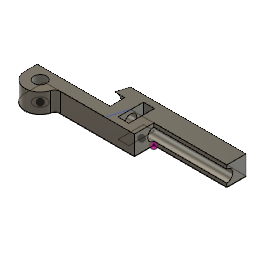
belt-tightener (Autodesk Fusion 360 design; units mm, degrees)
Autodesk Fusion 360 part; units mm, degrees
note: some values were not read from the file. Set by a fixed rule: which sketch regions a step uses.
sketch "Sketch1" plane through (0, 0, 0) normal (0, 1, 0) x (1, 0, 0)
  line L0 (12, 3.2) -> (12, 0)
  line L1 (12, 0) -> (0, 0)
  line L2 (-18, -3.2) -> (-18, 0)
  circle A0 centre (-15.5, -3.2) radius 1.05
  line L3 (-7.0785, 3.2) -> (-8, 0)
  line L4 (-8, 0) -> (-18, 0)
  line L5 (-7.0785, 3.2) -> (12, 3.2)
  line L6 (-3.8, 2.1) -> (-3.8, -2.1)
  line L7 (-3.8, -2.1) -> (-2, -2.1)
  line L8 (-2, -2.1) -> (-2, 2.1)
  line L9 (-2, 2.1) -> (-3.8, 2.1)
  line L10 (0, -3.2) -> (-13, -3.2)
  line L11 (0, -3.2) -> (0, 0)
  arc A1 (-18, -3.2) -> (-13, -3.2) centre (-15.5, -3.2) ccw
  dimension "d9" = 2.1
  dimension "d15" = 3.2
  dimension "d22" = 10
  dimension "d23" = 4.2
  dimension "d24" = 1.8
  dimension "d35" = 12
  dimension "d37" = 2.5
  dimension "d39" = 3.2
  dimension "d40" = 18
  dimension "d42" = 5
  dimension "d43" = 3.2
  dimension "d50" = 2
  measures "d9" diameter of A0
  measures "d35" distance of L1.end
  measures "d37" distance of L2
  measures "d39" distance of L1.end
  measures "d40" distance of L2 L11
  measures "d42" distance of L2
  measures "d50" distance of L1.end
extrude "Extrude2" add sketch "Sketch1" along normal blind 3.2
sketch "Sketch3" plane through (-18, 0, 0) normal (-1, 0, 0) x (0, 0, 1)
  line L0 (0, 0) -> (3.2, 0)
  line L1 (3.2, 0) -> (3.2, 3.2)
  line L2 (3.2, 3.2) -> (0, 3.2)
  line L3 (0, 3.2) -> (0, 0)
  circle A0 centre (0, 1.6) radius 1
  circle A1 centre (0, 1.6) radius 2
  dimension "d44" = 2
  dimension "d45" = 4
  measures "d44" diameter of A0
  measures "d45" diameter of A1
extrude "Extrude7" cut sketch "Sketch3" against normal blind 30 contours L3 A0 | L3 A0
extrude "Extrude8" cut sketch "Sketch3" against normal blind 12 contours L0 L2 L3 A0 A1 | L0 L2 L3 A0 A1
fillet "Fillet4" radius 1 1 edges at (-13, 1.6, 3.2)
